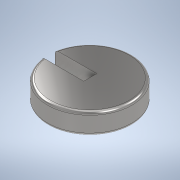
# Autodesk Inventor part: Hammer
Saved by Autodesk Inventor 2020 (Build 240168000, 168)
## iProperties
Created: 2021-12-24
Part Number: Hammer
Material: Iron, Malleable
Document SubType Name: Modeling
Designer: Umur Batuhan Özmen
Density: 7.15 g/cm^3
Appearance: Semi-Polished
Author: Umur Batuhan Özmen
Autodesk Inventor part; units mm, degrees
ref_plane "YZ Plane" through (0, 0, 0) normal (1, 0, 0) x (0, 1, 0)
ref_plane "XZ Plane" through (0, 0, 0) normal (0, 1, 0) x (-1, 0, 0)
ref_plane "XY Plane" through (0, 0, 0) normal (0, 0, 1) x (1, 0, 0)
sketch "Sketch1" plane through (0, 0, 0) normal (0, 1, 0) x (-1, 0, 0)
  arc A0 (29.684, 4.343) -> (29.5804, -5) centre (0, 0) ccw
  line L0 (29.5804, -5) -> (0, -5)
  line L1 (0, -5) -> (0, 4.343)
  line L2 (0, 4.343) -> (29.684, 4.343)
  dimension "d0" = 60
  constraints: 6 end point, 2 perpendicular, 2 point on circle, 1 centre point, 1 coincident
  measures "d0" diameter of A0
extrude "Extrusion1" add sketch "Sketch1" along normal blind 15
fillet "Fillet1" radius 2 2 edges at (29.9982, 15, 0.3325) (29.9982, 0, 0.3325)
body "Solid1"
